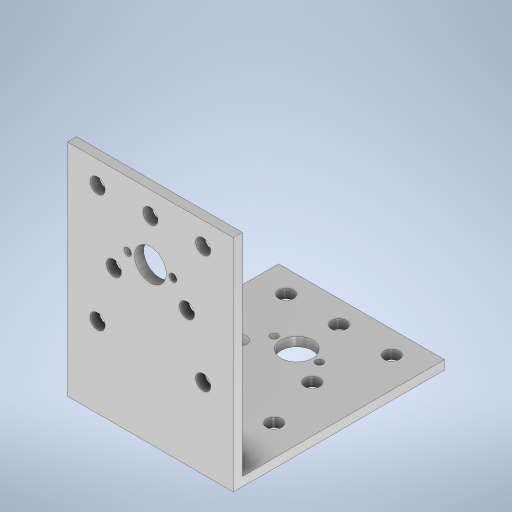
# Autodesk Inventor part: Metal Braket
Saved by Autodesk Inventor 2024 (Build 280153000, 153)
## iProperties
Created: 2023-07-17
Part Number: Metal Braket
Material: Aluminum 6061
Document SubType Name: Modeling
Designer: javie
Density: 2.7 g/cm^3
Appearance: Aluminum - Dark
Author: javie
Autodesk Inventor part; units mm, degrees
ref_plane "YZ Plane" through (0, 0, 0) normal (1, 0, 0) x (0, 1, 0)
ref_plane "XZ Plane" through (0, 0, 0) normal (0, 1, 0) x (-1, 0, 0)
ref_plane "Work Plane1" through (218.6643, -82.569, 72.5272) normal (0, 0, 1) x (1, 0, 0)
sketch "Sketch1" plane through (218.6643, -82.569, 72.5272) normal (0, 0, 1) x (1, 0, 0)
  line L0 (17.0344, 125.1412) -> (87.0344, 125.1412)
  line L1 (87.0344, 125.1412) -> (87.0344, 70.1412)
  line L2 (87.0344, 70.1412) -> (17.0344, 70.1412)
  line L3 (17.0344, 70.1412) -> (17.0344, 125.1412)
  point P0 (-218.6643, 82.569)
  dimension "Floor_Len" = 70
  dimension "Floor_Wid" = 55
  constraints: 8 end point, 2 parallel, 1 horizontal, 1 perpendicular
  measures "Floor_Len" distance of L1.end L2.end
  measures "Floor_Wid" distance of L0.end L1.end
extrude "Extrusion1" add sketch "Sketch1" along normal blind 3
sketch "Sketch2" plane through (218.6643, -82.569, 75.5272) normal (0, 0, 1) x (1, 0, 0)
  line L0 (17.0344, 70.1412) -> (87.0344, 70.1412) projected
  line L1 (87.0344, 125.1412) -> (17.0344, 125.1412) projected
  line L2 (87.0344, 70.1412) -> (84.0344, 70.1412)
  line L3 (84.0344, 70.1412) -> (84.0344, 125.1412)
  line L4 (84.0344, 125.1412) -> (87.0344, 125.1412)
  line L5 (87.0344, 125.1412) -> (87.0344, 70.1412)
  point P0 (-218.6643, 82.569)
  dimension "Tall_Thick" = 3
  constraints: 8 end point, 2 parallel, 1 horizontal, 1 perpendicular, 1 point on line
  measures "Tall_Thick" distance of L3.end L4.end
extrude "Extrusion2" add sketch "Sketch2" along normal blind 70
sketch "Sketch3" plane through (305.6987, -12.4279, 72.5272) normal (1, 0, 0) x (0, 0, -1)
  line L0 (0, 55) -> (-73, 55) projected
  line L1 (-73, 0) -> (-73, 55) projected
  point P0 (72.5272, 12.4279)
  point P1 (-51.5, 27.5)
  dimension "d40" = 21.5
  dimension "d41" = 27.5
  measures "d40" distance from line of L1 point (-51.5, 27.5)
  measures "d41" distance from line of L0 point (-51.5, 27.5)
hole "Hole1" at (305.6987, 15.0721, 124.0272) direction (-1, 0, 0) diameter 10.5 end through all
sketch "Sketch4" plane through (305.6987, -12.4279, 72.5272) normal (1, 0, 0) x (0, 0, -1)
  circle A0 centre (-51.5, 27.5) radius 5.3956
  circle A1 centre (-51.5, 27.5) radius 5.25 projected
  point P0 (72.5272, 12.4279)
  point P1 (-51.5, 20)
  point P2 (-51.5, 35)
  dimension "d46" = 7.5
  dimension "d47" = 7.5
  constraints: 2 vertical alignment, 1 centre point, 1 concentric
  measures "d46" distance of point (-51.5, 20) A0.centre
  measures "d47" distance of A0.centre point (-51.5, 35)
hole "Hole2" at (305.6987, 7.5721, 124.0272) at (305.6987, 22.5721, 124.0272) direction (-1, 0, 0) diameter 2.5 end through all
sketch "Sketch5" plane through (305.6987, -12.4279, 72.5272) normal (1, 0, 0) x (0, 0, -1)
  circle A0 centre (-51.5, 27.5) radius 5.2922
  circle A1 centre (-51.5, 27.5) radius 5.25 projected
  line L0 (-65.5, 27.5) -> (-44.5, 39.6244)
  line L1 (-44.5, 39.6244) -> (-44.5, 15.3756)
  line L2 (-44.5, 15.3756) -> (-65.5, 27.5)
  point P0 (-65.5, 10)
  point P1 (-65.5, 45)
  point P2 (-26.5, 10)
  point P3 (-26.5, 45)
  dimension "d42" = 14
  dimension "d43" = 17.5
  dimension "d44" = 17.5
  dimension "d45" = 39
  constraints: 6 end point, 3 coincident, 3 horizontal alignment, 3 vertical alignment, 1 centre point, 1 concentric, 7 other
  measures "d42" distance of A0.centre L0.start
  measures "d43" distance of point (-65.5, 10) L0.start
  measures "d44" distance of point (-65.5, 45) L0.start
  measures "d45" distance of point (-26.5, 45) point (-65.5, 45)
hole "Hole3" at (305.6987, -2.4279, 138.0272) at (305.6987, -2.4279, 99.0272) at (305.6987, 32.5721, 99.0272) at (305.6987, 32.5721, 138.0272) at (305.6987, 15.0721, 138.0272) at (305.6987, 2.9478, 117.0272) at (305.6987, 27.1965, 117.0272) direction (-1, 0, 0) diameter 5 end through all
sketch "Sketch6" plane through (242.6987, 66.5721, 72.5272) normal (0, 0, -1) x (0, 1, 0)
  line L0 (-24, -7) -> (-79, -7) projected
  line L1 (-24, 63) -> (-24, -7) projected
  point P0 (72.5272, 12.4279)
  point P1 (-51.5, 14.5)
  dimension "d77" = 21.5
  dimension "d78" = 27.5
  measures "d77" distance from line of L0 point (-51.5, 14.5)
  measures "d78" distance from line of L1 point (-51.5, 14.5)
hole "Hole4" at (257.1987, 15.0721, 72.5272) direction (0, 0, 1) diameter 10.5 end through all
sketch "Sketch7" plane through (270.6987, 15.0721, 72.5272) normal (0, 0, -1) x (-1, 0, 0)
  circle A0 centre (13.5, 0) radius 5.3956
  circle A1 centre (13.5, 0) radius 5.25 projected
  point P0 (72.5272, 12.4279)
  point P1 (13.5, -7.5)
  point P2 (13.5, 7.5)
  dimension "d59" = 7.5
  dimension "d58" = 7.5
  constraints: 2 vertical alignment, 1 centre point, 1 concentric
  measures "d59" distance of point (13.5, -7.5) A0.centre
  measures "d58" distance of A0.centre point (13.5, 7.5)
hole "Hole5" at (257.1987, 7.5721, 72.5272) at (257.1987, 22.5721, 72.5272) direction (0, 0, 1) diameter 2.5 end through all
sketch "Sketch8" plane through (270.6987, 15.0721, 72.5272) normal (0, 0, -1) x (-1, 0, 0)
  line L0 (35, -27.5) -> (-32, -27.5) projected
  circle A0 centre (13.5, 0) radius 5.25
  circle A1 centre (13.5, 0) radius 5.25 projected
  line L1 (27.5, 0) -> (6.5, -12.1244)
  line L2 (6.5, -12.1244) -> (6.5, 12.1244)
  line L3 (6.5, 12.1244) -> (27.5, 0)
  point P0 (27.5, 17.5)
  point P1 (27.5, -17.5)
  point P2 (-11.5, 17.5)
  point P3 (-11.5, -17.5)
  dimension "d79" = 17.5
  dimension "d80" = 17.5
  dimension "d82" = 39
  dimension "d83" = 10
  dimension "d84" = 10.5
  dimension "d85" = 14
  constraints: 6 end point, 3 coincident, 3 vertical alignment, 2 horizontal alignment, 1 centre point, 1 concentric, 7 other
  measures "d79" distance of point (27.5, -17.5) L1.start
  measures "d80" distance of L1.start point (27.5, 17.5)
  measures "d82" distance of point (-11.5, 17.5) point (27.5, 17.5)
  measures "d83" distance from line of L0 point (27.5, -17.5)
  measures "d84" diameter of A0
  measures "d85" distance of A0.centre L1.start
hole "Hole6" at (243.1987, 15.0721, 72.5272) at (243.1987, 32.5721, 72.5272) at (282.1987, 32.5721, 72.5272) at (282.1987, -2.4279, 72.5272) at (243.1987, -2.4279, 72.5272) at (264.1987, 27.1965, 72.5272) at (264.1987, 2.9478, 72.5272) direction (0, 0, 1) diameter 5 end through all
equation "\"d41\" = 0.5 * Floor_Wid"
equation "\"d78\" = 0.5 * Floor_Wid"
body "Solid1"
